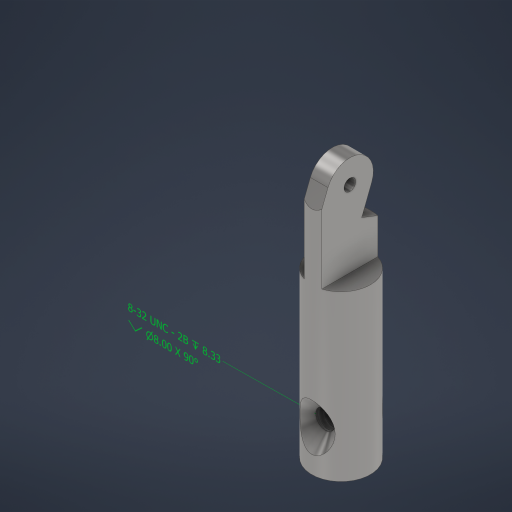
# Autodesk Inventor part: barrel_hinge-male
Saved by Autodesk Inventor 2023 (Build 270158000, 158)
## iProperties
Created: 2022-04-23
Part Number: barrel_hinge-male
Material: Stainless Steel
Document SubType Name: Modeling
Designer: Norbert Ligas
Density: 8 g/cm^3
Appearance: Semi-Polished
Author: Norbert Ligas
Autodesk Inventor part; units mm, degrees
ref_plane "XZ Plane" through (0, 0, 0) normal (0, 1, 0) x (-1, 0, 0)
sketch "Sketch1" plane through (0, 0, 0) normal (0, 1, 0) x (-1, 0, 0)
  circle A0 centre (0, 0) radius 5
  dimension "d0" = 10
  constraints: 1 centre point, 1 coincident
  measures "d0" diameter of A0
extrude "Extrusion1" add sketch "Sketch1" along normal blind 45
ref_plane "Work Plane1" through (0, 0, 5) normal (0, 0, 1) x (1, 0, 0)
sketch "Sketch2" plane through (0, 0, 5) normal (0, 0, 1) x (1, 0, 0)
  point P0 (0, 0)
  point P1 (0, 7)
  dimension "d3" = 7
  constraints: 1 vertical alignment
  measures "d3" distance of point (0, 0) point (0, 7)
hole "Hole1" at (0, 7, 5) direction (0, 0, -1) diameter 3.302 end through all countersink diameter 8 countersink angle 90 thread size "8-32 UNC" class "2B" standard "ANSI Unified Screw Threads"
sketch "Sketch5" plane through (0, 45, 0) normal (0, 1, 0) x (1, 0, 0)
  line L0 (-5, 5) -> (-1.5, 5)
  line L1 (-1.5, 5) -> (-1.5, -5)
  line L2 (-1.5, -5) -> (-5, -5)
  line L3 (-5, -5) -> (-5, 5)
  line L4 (1.5, 5) -> (5, 5)
  line L5 (5, 5) -> (5, -5)
  line L6 (5, -5) -> (1.5, -5)
  line L7 (1.5, -5) -> (1.5, 5)
  point P0 (0, 0)
  point P1 (-5, 0)
  point P2 (1.5, 0)
  point P3 (5, 0)
  point P4 (-1.5, 0)
  dimension "d16" = 3
  dimension "d17" = 10
  dimension "d18" = 10
  dimension "d27" = 5
  constraints: 16 end point, 12 horizontal alignment, 4 midpoint, 4 parallel, 2 horizontal, 2 perpendicular, 1 collinear, 1 point on line
  measures "d16" distance of L6.end L1.end
  measures "d17" distance of L5.end L2.end
  measures "d18" distance of L5.end L4.end
  measures "d27" horizontal distance of point (0, 0) L4.end
extrude "Extrusion2" cut sketch "Sketch5" against normal blind 17
sketch "Sketch6" plane through (1.5, 45, 4.7697) normal (1, 0, 0) x (0, 0, -1)
  circle A0 centre (4.7697, -4) radius 1
  line L0 (0, 0) -> (9.5394, 0) projected
  line L1 (0, -17) -> (0, 0) projected
  line L2 (0, -17) -> (9.5394, -17) projected
  line L3 (9.5394, 0) -> (0, 0) projected
  line L4 (9.5394, 0) -> (9.5394, -17) projected
  line L5 (4.7697, 0) -> (4.7697, -17)
  point P0 (4.7697, -45)
  dimension "d32" = 2
  dimension "d33" = 4
  constraints: 2 end point, 2 midpoint, 1 centre point, 1 point on line
  measures "d32" diameter of A0
  measures "d33" distance from line of L0 A0.centre
hole "Hole2" at (1.5, 41, 0) direction (-1, 0, 0) diameter 2 end through all
ref_plane "Work Plane3" through (5, 0, 0) normal (1, 0, 0) x (0, 1, 0)
sketch "Sketch10" plane through (5, 0, 0) normal (1, 0, 0) x (0, 1, 0)
  arc A0 (39.5485, -3.7274) -> (45, 0) centre (41, 0) ccw
  circle A1 centre (41, 0) radius 1 projected
  line L0 (28, 0.7697) -> (39.5485, -3.7274)
  line L1 (28, 4.7697) -> (28, -4.7697) projected
  line L2 (28, 4.7697) -> (45, 4.7697) projected
  line L3 (45, -5) -> (45, -4.7697) projected
  line L4 (34, -5) -> (45, -5)
  line L5 (45, 4.7697) -> (45, 5) projected
  line L6 (45, -5) -> (45, 5)
  line L7 (45, 5) -> (39.1833, 5)
  line L8 (39.1833, 5) -> (42.4515, 3.7274)
  line L9 (45, 4.7697) -> (28, 4.7697) projected
  line L10 (0, 5) -> (45, 5) projected
  line L11 (34, -5) -> (35.1609, -2.0188)
  arc A2 (45, 0) -> (42.4515, 3.7274) centre (41, 0) ccw
  point P0 (0, 0)
  point P1 (45, -4.7697)
  dimension "d54" = 8
  dimension "d55" = 6
  dimension "d56" = 4
  constraints: 12 end point, 4 point on circle, 4 tangent, 3 point on line, 2 centre point, 2 perpendicular, 1 coincident, 1 collinear, 1 horizontal, 1 midpoint
  measures "d54" diameter of A0
  measures "d55" horizontal distance of L1.end L4.start
  measures "d56" distance from line of L2 L0.start
extrude "Extrusion3" cut sketch "Sketch10" against normal through all contours A0 L6 L3 L4 L11 L0 | A2 L8 L2 L6 | L2 L8 L7 L5
chamfer "Chamfer1" distance 2 angle 45 1 edges at (-0.2563, 8.631, -4.9934)
